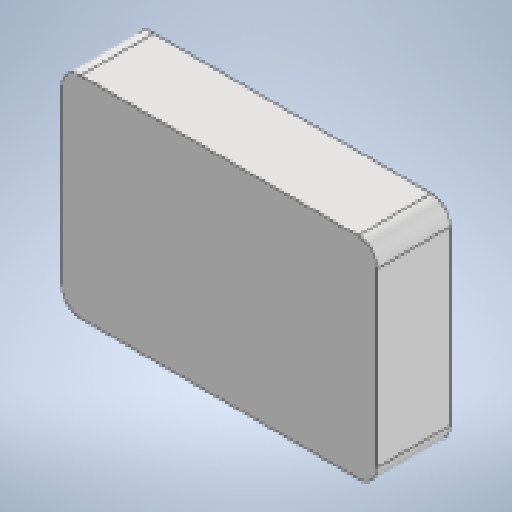
# Autodesk Inventor part: shell_bttm
Saved by Autodesk Inventor 2025.1 (Build 291241000, 241)
## iProperties
Created: 2025-05-05
Part Number: shell_bttm
Material: Generic
Document SubType Name: Modeling
Designer: santiago
Density: 1 g/cm^3
Appearance: Default
Author: santiago
Autodesk Inventor part; units mm, degrees
ref_plane "YZ Plane" through (0, 0, 0) normal (1, 0, 0) x (0, 1, 0)
ref_plane "XZ Plane" through (0, 0, 0) normal (0, 1, 0) x (-1, 0, 0)
ref_plane "XY Plane" through (0, 0, 0) normal (0, 0, 1) x (1, 0, 0)
sketch "Sketch1" plane through (0, 0, 0) normal (0, 0, 1) x (1, 0, 0)
  arc A0 (41.25, 22.5) -> (36.25, 27.5) centre (36.25, 22.5) ccw projected
  line L0 (36.25, 27.5) -> (-36.25, 27.5) projected
  arc A1 (-36.25, 27.5) -> (-41.25, 22.5) centre (-36.25, 22.5) ccw projected
  line L1 (-41.25, 22.5) -> (-41.25, -22.5) projected
  arc A2 (-41.25, -22.5) -> (-36.25, -27.5) centre (-36.25, -22.5) ccw projected
  line L2 (-36.25, -27.5) -> (36.25, -27.5) projected
  arc A3 (36.25, -27.5) -> (41.25, -22.5) centre (36.25, -22.5) ccw projected
  line L3 (41.25, -22.5) -> (41.25, 22.5) projected
  line L4 (36.25, -25.5) -> (-36.25, -25.5) projected
  arc A4 (-39.25, -22.5) -> (-36.25, -25.5) centre (-36.25, -22.5) ccw projected
  line L5 (-39.25, -22.5) -> (-39.25, 22.5) projected
  arc A5 (-36.25, 25.5) -> (-39.25, 22.5) centre (-36.25, 22.5) ccw projected
  line L6 (-36.25, 25.5) -> (36.25, 25.5) projected
  arc A6 (39.25, 22.5) -> (36.25, 25.5) centre (36.25, 22.5) ccw projected
  line L7 (39.25, 22.5) -> (39.25, -22.5) projected
  arc A7 (36.25, -25.5) -> (39.25, -22.5) centre (36.25, -22.5) ccw projected
  point P0 (0, 0)
extrude "Extrusion1" add sketch "Sketch1" along normal blind 22.5
sketch "Sketch2" plane through (0, 0, 22.5) normal (0, 0, 1) x (1, 0, 0)
  line L0 (-36.25, 25.5) -> (36.25, 25.5) projected
  arc A0 (-36.25, 25.5) -> (-39.25, 22.5) centre (-36.25, 22.5) ccw projected
  line L1 (-39.25, -22.5) -> (-39.25, 22.5) projected
  arc A1 (-39.25, -22.5) -> (-36.25, -25.5) centre (-36.25, -22.5) ccw projected
  line L2 (36.25, -25.5) -> (-36.25, -25.5) projected
  arc A2 (36.25, -25.5) -> (39.25, -22.5) centre (36.25, -22.5) ccw projected
  line L3 (39.25, 22.5) -> (39.25, -22.5) projected
  arc A3 (39.25, 22.5) -> (36.25, 25.5) centre (36.25, 22.5) ccw projected
  point P0 (0, 0)
extrude "Extrusion2" add sketch "Sketch2" against normal blind 2
sketch "Sketch3" plane through (0, 0, 20.5) normal (0, 0, -1) x (-1, 0, 0)
  arc A0 (39.25, 22.5) -> (36.25, 25.5) centre (36.25, 22.5) ccw projected
  line L0 (39.25, 22.5) -> (39.25, 19.5) projected
  line L1 (39.25, 19.5) -> (36.25, 19.5) projected
  arc A1 (33.25, 22.5) -> (36.25, 19.5) centre (36.25, 22.5) ccw projected
  line L2 (33.25, 22.5) -> (33.25, 25.5) projected
  line L3 (33.25, 25.5) -> (36.25, 25.5) projected
  circle A2 centre (36.25, 22.5) radius 2.25 projected
  circle A3 centre (36.25, -22.5) radius 2.25 projected
  arc A4 (36.25, -25.5) -> (39.25, -22.5) centre (36.25, -22.5) ccw projected
  line L4 (36.25, -25.5) -> (33.25, -25.5) projected
  line L5 (33.25, -25.5) -> (33.25, -22.5) projected
  arc A5 (36.25, -19.5) -> (33.25, -22.5) centre (36.25, -22.5) ccw projected
  line L6 (36.25, -19.5) -> (39.25, -19.5) projected
  line L7 (39.25, -19.5) -> (39.25, -22.5) projected
  arc A6 (-39.25, -22.5) -> (-36.25, -25.5) centre (-36.25, -22.5) ccw projected
  line L8 (-39.25, -22.5) -> (-39.25, -19.5) projected
  line L9 (-39.25, -19.5) -> (-36.25, -19.5) projected
  arc A7 (-33.25, -22.5) -> (-36.25, -19.5) centre (-36.25, -22.5) ccw projected
  line L10 (-33.25, -22.5) -> (-33.25, -25.5) projected
  line L11 (-33.25, -25.5) -> (-36.25, -25.5) projected
  circle A8 centre (-36.25, -22.5) radius 2.25 projected
  arc A9 (-36.25, 25.5) -> (-39.25, 22.5) centre (-36.25, 22.5) ccw projected
  line L12 (-36.25, 25.5) -> (-33.25, 25.5) projected
  line L13 (-33.25, 25.5) -> (-33.25, 22.5) projected
  arc A10 (-36.25, 19.5) -> (-33.25, 22.5) centre (-36.25, 22.5) ccw projected
  line L14 (-36.25, 19.5) -> (-39.25, 19.5) projected
  line L15 (-39.25, 19.5) -> (-39.25, 22.5) projected
  circle A11 centre (-36.25, 22.5) radius 2.25 projected
  circle A12 centre (-36.25, 22.5) radius 1.7
  circle A13 centre (-36.25, -22.5) radius 1.7
  circle A14 centre (36.25, -22.5) radius 1.7
  circle A15 centre (36.25, 22.5) radius 1.7
  point P0 (0, 0)
  dimension "d4" = 3.4
  dimension "d5" = 3.4
  dimension "d6" = 3.4
  dimension "d7" = 3.4
  constraints: 4 centre point, 4 coincident
  measures "d4" diameter of A12
  measures "d5" diameter of A15
  measures "d6" diameter of A13
  measures "d7" diameter of A14
ref_plane "Work Plane1" through (33.25, 19.5, 10) normal (0, 0, 1) x (1, 0, 0)
extrude "Extrusion3" add sketch "Sketch3" along normal up to surface (10.5 mm away) contours L0 L1 A1 L2 L3 A0 | A2 | A3 | L4 L5 A5 L6 L7 A4 | L8 L9 A7 L10 L11 A6 | A8 | L12 L13 A10 L14 L15 A9 | A11
sketch "Sketch4" plane through (0, 0, 22.5) normal (0, 0, 1) x (1, 0, 0)
  circle A0 centre (-36.25, 22.5) radius 1.7 projected
  circle A1 centre (36.25, 22.5) radius 1.7 projected
  circle A2 centre (36.25, -22.5) radius 1.7 projected
  circle A3 centre (-36.25, -22.5) radius 1.7 projected
  point P0 (0, 0)
extrude "Extrusion4" cut sketch "Sketch4" against normal blind 22.5
fillet "Fillet1" radius 3 8 edges at (-39.7855, 26.0355, 22.5) (-41.25, 0, 22.5) (-39.7855, -26.0355, 22.5) (0, -27.5, 22.5) (39.7855, -26.0355, 22.5) (41.25, 0, 22.5) (39.7855, 26.0355, 22.5) (0, 27.5, 22.5)
sketch "Sketch5" plane through (0, 0, 22.5) normal (0, 0, 1) x (1, 0, 0)
  circle A0 centre (-36.25, 22.5) radius 1.7 projected
  circle A1 centre (-36.25, 22.5) radius 2.45
  circle A2 centre (36.25, 22.5) radius 1.7 projected
  circle A3 centre (36.25, 22.5) radius 2.45
  circle A4 centre (-36.25, -22.5) radius 1.7 projected
  circle A5 centre (-36.25, -22.5) radius 2.45
  circle A6 centre (36.25, -22.5) radius 1.7 projected
  circle A7 centre (36.25, -22.5) radius 2.45
  point P0 (0, 0)
  dimension "d13" = 4.9
  dimension "d14" = 4.9
  dimension "d15" = 4.9
  dimension "d16" = 4.9
  constraints: 4 centre point, 4 coincident
  measures "d13" diameter of A1
  measures "d14" diameter of A3
  measures "d15" diameter of A5
  measures "d16" diameter of A7
extrude "Extrusion5" cut sketch "Sketch5" against normal blind 2 contours A0 | A1 | A2 | A3 | A4 | A5 | A6 | A7
fillet "Fillet2" radius 3 4 edges at (0, 25.5, 20.5) (39.25, 0, 20.5) (0, -25.5, 20.5) (-39.25, 0, 20.5)
fillet "Fillet3" radius 1 20 edges at (-33.25, 24.6213, 19.6213) (-34.1287, 20.3787, 20.5) (-38.3713, 19.5, 19.6213) (-39.25, 19.5, 13.75) (-33.25, 25.5, 13.75) (33.25, 24.6213, 19.6213) (34.1287, 20.3787, 20.5) (38.3713, 19.5, 19.6213) (39.25, 19.5, 13.75) (33.25, 25.5, 13.75) (33.25, -24.6213, 19.6213) (33.25, -25.5, 13.75) (38.3713, -19.5, 19.6213) (39.25, -19.5, 13.75) (34.1287, -20.3787, 20.5) (-38.3713, -19.5, 19.6213) (-39.25, -19.5, 13.75) (-33.25, -24.6213, 19.6213) (-33.25, -25.5, 13.75) (-34.1287, -20.3787, 20.5)
sketch "Sketch6" plane through (0, 0, 22.5) normal (0, 0, 1) x (1, 0, 0)
  line L0 (-34.8349, 24.5) -> (34.8349, 24.5) projected
  line L1 (38.25, 21.0849) -> (38.25, -21.0849) projected
  line L2 (-6.55, 0) -> (6.55, 0) construction
  line L3 (-4.5, -2.05) -> (4.5, -2.05)
  line L4 (4.5, 2.05) -> (-4.5, 2.05)
  arc A0 (-4.5, 2.05) -> (-4.5, -2.05) centre (-4.5, 0) ccw
  arc A1 (4.5, -2.05) -> (4.5, 2.05) centre (4.5, 0) ccw
  point P0 (0, 0)
  point P1 (0, 0)
  point P2 (0, 2.05)
  dimension "d21" = 13.1
  dimension "d22" = 4.1
  constraints: 8 end point, 6 point on circle, 4 tangent, 2 centre point, 2 midpoint, 2 point on line, 1 horizontal, 1 parallel, 1 vertical alignment
  measures "d21" distance of L2.start L2.end
  measures "d22" diameter of A1
extrude "Extrusion6" cut sketch "Sketch6" against normal through all
sketch "Sketch7" plane through (0, 0, 22.5) normal (0, 0, 1) x (1, 0, 0)
  line L0 (-4.5, 2.05) -> (4.5, 2.05) projected
  arc A0 (4.5, -2.05) -> (4.5, 2.05) centre (4.5, 0) ccw projected
  line L1 (4.5, -2.05) -> (-4.5, -2.05) projected
  arc A1 (-4.5, 2.05) -> (-4.5, -2.05) centre (-4.5, 0) ccw projected
  line L2 (-9.375, 0) -> (9.375, 0) construction
  line L3 (-7.325, -2.05) -> (7.325, -2.05)
  line L4 (7.325, 2.05) -> (-7.325, 2.05)
  arc A2 (-7.325, 2.05) -> (-7.325, -2.05) centre (-7.325, 0) ccw
  arc A3 (7.325, -2.05) -> (7.325, 2.05) centre (7.325, 0) ccw
  point P0 (0, 0)
  point P1 (0, 0)
  point P2 (4.5, -2.05)
  dimension "d25" = 18.75
  dimension "d26" = 4.1
  constraints: 8 end point, 6 point on circle, 4 tangent, 2 centre point, 2 point on line, 1 coincident, 1 horizontal, 1 midpoint, 1 parallel
  measures "d25" distance of L2.start L2.end
  measures "d26" diameter of A3
extrude "Extrusion7" add sketch "Sketch7" against normal blind 2.1 contours A1 L3 A2 L4 | L4 A3 L3 A0
sketch "Sketch8" plane through (0, 0, 22.5) normal (0, 0, 1) x (1, 0, 0)
  line L0 (-11.375, 0) -> (11.375, 0) construction
  line L1 (-7.325, -4.05) -> (7.325, -4.05)
  line L2 (7.325, 4.05) -> (-7.325, 4.05)
  arc A0 (-7.325, 4.05) -> (-7.325, -4.05) centre (-7.325, 0) ccw
  arc A1 (7.325, -4.05) -> (7.325, 4.05) centre (7.325, 0) ccw
  line L3 (-4.5, 2.05) -> (4.5, 2.05) projected
  arc A2 (-4.5, 2.05) -> (-4.5, -2.05) centre (-4.5, 0) ccw projected
  line L4 (4.5, -2.05) -> (-4.5, -2.05) projected
  arc A3 (4.5, -2.05) -> (4.5, 2.05) centre (4.5, 0) ccw projected
  arc A4 (-7.325, 2.05) -> (-7.325, -2.05) centre (-7.325, 0) ccw projected
  line L5 (-4.5, 2.05) -> (-7.325, 2.05) projected
  line L6 (-7.325, -2.05) -> (-4.5, -2.05) projected
  line L7 (7.325, 2.05) -> (4.5, 2.05) projected
  arc A5 (7.325, -2.05) -> (7.325, 2.05) centre (7.325, 0) ccw projected
  line L8 (4.5, -2.05) -> (7.325, -2.05) projected
  point P0 (0, 0)
  point P1 (0, 0)
  point P2 (0, 4.05)
  dimension "d29" = 22.75
  dimension "d30" = 8.1
  constraints: 8 end point, 6 point on circle, 4 tangent, 2 centre point, 2 midpoint, 2 point on line, 1 horizontal, 1 parallel, 1 vertical alignment
  measures "d29" distance of L0.start L0.end
  measures "d30" diameter of A1
extrude "Extrusion8" add sketch "Sketch8" against normal blind 2.9
equation "\"d5\" = d4"
equation "\"d6\" = d4"
equation "\"d7\" = d4"
body "Solid1"
